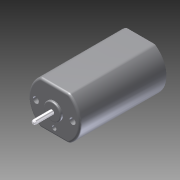
# Autodesk Inventor part: QFK-N30QAV-16068
Saved by Autodesk Inventor 2013 (Build 170138000, 138)
## iProperties
Category: Motoors
Company: Autodesk Inc.
Created: 2012-01-24
Part Number: QFK-N30QAV-16068
Material: Generic
Document SubType Name: Modeling
Designer: Autodesk Inc.
Density: 1 g/cm^3
Catalog Web Link: http://www.vexrobotics.com/276-2181.html
Vendor: VEX
Author: Autodesk Inc.
Autodesk Inventor part; units mm, degrees
ref_plane "YZ Plane" through (0, 0, 0) normal (1, 0, 0) x (0, 1, 0)
ref_plane "XZ Plane" through (0, 0, 0) normal (0, 1, 0) x (-1, 0, 0)
ref_plane "XY Plane" through (0, 0, 0) normal (0, 0, 1) x (1, 0, 0)
sketch "Sketch1" plane through (0, 0, 0) normal (0, 0, 1) x (1, 0, 0)
  line L0 (-3.0031, 5) -> (3.0031, 5)
  arc A0 (-3.597, 4.8023) -> (-3.6, -4.8) centre (0, 0) ccw
  line L1 (3.0031, -5) -> (-3.0031, -5)
  arc A1 (-3.597, 4.8023) -> (-3.597, -4.8023) centre (0, 0) ccw
  arc A2 (3.597, -4.8023) -> (3.597, 4.8023) centre (0, 0) ccw
  arc A3 (-3.0031, 5) -> (-3.597, 4.8023) centre (-3.0031, 4.0094) ccw
  arc A4 (3.597, 4.8023) -> (3.0031, 5) centre (3.0031, 4.0094) ccw
  arc A5 (3.0031, -5) -> (3.597, -4.8023) centre (3.0031, -4.0094) ccw
  arc A6 (-3.597, -4.8023) -> (-3.0031, -5) centre (-3.0031, -4.0094) ccw
  point P0 (0, 0)
  point P1 (3.3166, 5)
  point P2 (3.3166, -5)
  point P3 (-3.3166, -5)
  dimension "d0" = 0.9906
  constraints: 18 point on circle, 8 tangent, 7 centre point, 4 end point, 3 equal radius, 3 point on line
  measures "d0" radius of A3
extrude "Extrusion1" add sketch "Sketch1" along normal mid plane 19.9898
fillet "Fillet1" radius 0.508 8 edges at (-3.3161, 4.9493, 9.9949) (-6, 0, 9.9949) (-3.3161, -4.9493, 9.9949) (0, -5, 9.9949) (3.3161, -4.9493, 9.9949) (6, 0, 9.9949) (3.3161, 4.9493, 9.9949) (0, 5, 9.9949)
sketch "Sketch2" plane through (0, 0, 9.9949) normal (0, 0, 1) x (1, 0, 0)
  arc A0 (-3, 4.5) -> (-3.3, 4.4) centre (-2.9981, 3.9944) ccw
  spline S0 degree 3 poles (-3.3, 4.4) (-3.4685, 4.2736) (-3.6287, 4.1385) (-3.7806, 3.9947) (-3.8945, 3.8869) (-4.0038, 3.7742) (-4.1084, 3.6566) (-4.1433, 3.6174) (-4.1767, 3.5788) (-4.2115, 3.5374) (-4.4897, 3.2063) (-4.726, 2.8465) (-4.9194, 2.4597) (-5.0886, 2.1212) (-5.2214, 1.7694) (-5.3178, 1.4041) (-5.3315, 1.3519) (-5.3449, 1.298) (-5.3568, 1.2467) (-5.4522, 0.837) (-5.5, 0.4207) (-5.5, 0) (-5.5, -0.3681) (-5.4635, -0.7323) (-5.3904, -1.0926) (-5.38, -1.144) (-5.3691, -1.1941) (-5.3568, -1.2467) (-5.2588, -1.6679) (-5.1127, -2.0729) (-4.9194, -2.4597) (-4.7502, -2.7981) (-4.5484, -3.1155) (-4.3139, -3.4117) (-4.2805, -3.4541) (-4.2453, -3.4972) (-4.2115, -3.5374) (-3.941, -3.8595) (-3.6373, -4.147) (-3.3, -4.4) knots 0 0 0 0 0.0625 0.0625 0.0625 0.109375 0.109375 0.109375 0.125 0.125 0.125 0.25 0.25 0.25 0.359375 0.359375 0.359375 0.375 0.375 0.375 0.5 0.5 0.5 0.609375 0.609375 0.609375 0.625 0.625 0.625 0.75 0.75 0.75 0.859375 0.859375 0.859375 0.875 0.875 0.875 1 1 1 1
  arc A1 (-3.3, -4.4) -> (-3, -4.5) centre (-2.9981, -3.9944) ccw
  line L0 (-3, -4.5) -> (3, -4.5)
  arc A2 (3, -4.5) -> (3.3, -4.4) centre (2.9981, -3.9944) ccw
  arc A3 (3.3, -4.4) -> (3.3, 4.4) centre (0, 0) ccw
  arc A4 (3.3, 4.4) -> (3, 4.5) centre (2.9981, 3.9944) ccw
  line L1 (3, 4.5) -> (-3, 4.5)
  circle A5 centre (-4.25, 0) radius 0.7
  circle A6 centre (4.25, 0) radius 0.7
  circle A7 centre (0, 0) radius 2
  circle A8 centre (0, -3.5) radius 0.5
  circle A9 centre (0, -3.5) radius 0.5
  circle A10 centre (-4.25, 0) radius 0.7
  circle A11 centre (4.25, 0) radius 0.7
  circle A12 centre (0, 0) radius 2
  line L2 (3, 4.5) -> (-3, 4.5)
  arc A13 (-3, 4.5) -> (-3.3, 4.4) centre (-2.9981, 3.9944) ccw
  spline S1 degree 3 poles (-3.3, 4.4) (-3.4685, 4.2736) (-3.6287, 4.1385) (-3.7806, 3.9947) (-3.8945, 3.8869) (-4.0038, 3.7742) (-4.1084, 3.6566) (-4.1433, 3.6174) (-4.1767, 3.5788) (-4.2115, 3.5374) (-4.4897, 3.2063) (-4.726, 2.8465) (-4.9194, 2.4597) (-5.0886, 2.1212) (-5.2214, 1.7694) (-5.3178, 1.4041) (-5.3315, 1.3519) (-5.3449, 1.298) (-5.3568, 1.2467) (-5.4522, 0.837) (-5.5, 0.4207) (-5.5, 0) (-5.5, -0.3681) (-5.4635, -0.7323) (-5.3904, -1.0926) (-5.38, -1.144) (-5.3691, -1.1941) (-5.3568, -1.2467) (-5.2588, -1.6679) (-5.1127, -2.0729) (-4.9194, -2.4597) (-4.7502, -2.7981) (-4.5484, -3.1155) (-4.3139, -3.4117) (-4.2805, -3.4541) (-4.2453, -3.4972) (-4.2115, -3.5374) (-3.941, -3.8595) (-3.6373, -4.147) (-3.3, -4.4) knots 0 0 0 0 0.0625 0.0625 0.0625 0.109375 0.109375 0.109375 0.125 0.125 0.125 0.25 0.25 0.25 0.359375 0.359375 0.359375 0.375 0.375 0.375 0.5 0.5 0.5 0.609375 0.609375 0.609375 0.625 0.625 0.625 0.75 0.75 0.75 0.859375 0.859375 0.859375 0.875 0.875 0.875 1 1 1 1
  arc A14 (-3.3, -4.4) -> (-3, -4.5) centre (-2.9981, -3.9944) ccw
  line L3 (-3, -4.5) -> (3, -4.5)
  arc A15 (3, -4.5) -> (3.3, -4.4) centre (2.9981, -3.9944) ccw
  arc A16 (3.3, -4.4) -> (3.3, 4.4) centre (0, 0) ccw
  arc A17 (3.3, 4.4) -> (3, 4.5) centre (2.9981, 3.9944) ccw
  line L4 (-3, 5) -> (3, 5)
  arc A18 (3.6, -4.8) -> (3.6, 4.8) centre (0, 0) ccw
  arc A19 (-3.6, 4.8) -> (-3.6, -4.8) centre (0, 0) ccw
  line L5 (3, -5) -> (-3, -5)
  arc A20 (-3, 5) -> (-3.6, 4.8) centre (-3, 4) ccw
  constraints: 26 point on circle, 21 centre point, 12 end point, 4 other
extrude "Extrusion2" add sketch "Sketch2" along normal blind 0.508 contours A7
fillet "Fillet2" radius 0.254 1 edges at (-2, 0, 10.5029)
extrude "Extrusion3" cut sketch "Sketch2" against normal blind 2.9972 contours A5 | A6 | A8
sketch "Sketch3" plane through (0, 0, 10.5029) normal (0, 0, 1) x (1, 0, 0)
  circle A0 centre (0, 0) radius 1.746 projected
  circle A1 centre (0, 0) radius 0.4953
  dimension "d9" = 0.9906
  constraints: 1 centre point, 1 coincident
  measures "d9" diameter of A1
extrude "Extrusion4" add sketch "Sketch3" along normal blind 4.4958 contours A1
fillet "Fillet3" radius 0.4953 1 edges at (-0.4953, 0, 14.9987)
sketch "Sketch4" plane through (0, 0, -9.9949) normal (0, 0, -1) x (-1, 0, 0)
  arc A0 (-3.597, 4.8023) -> (-3.597, -4.8023) centre (0, 0) ccw projected
  circle A1 centre (0, 0) radius 2.5019
  dimension "d13" = 5.0038
  constraints: 1 centre point, 1 coincident
  measures "d13" diameter of A1
extrude "Extrusion5" add sketch "Sketch4" along normal blind 1.1938
sketch "Sketch5" plane through (0, 0, -9.9949) normal (0, 0, -1) x (-1, 0, 0)
  arc A0 (-3, 5) -> (-3.6, 4.8) centre (-3, 4) ccw
  arc A1 (-3.6, 4.8) -> (-3.6, -4.8) centre (0, 0) ccw
  arc A2 (-3.6, -4.8) -> (-3, -5) centre (-3, -4) ccw
  line L0 (3, -5) -> (-3, -5)
  arc A3 (3, -5) -> (3.6, -4.8) centre (3, -4) ccw
  arc A4 (3.6, -4.8) -> (3.6, 4.8) centre (0, 0) ccw
  arc A5 (3.6, 4.8) -> (3, 5) centre (3, 4) ccw
  line L1 (-3, 5) -> (3, 5)
  line L2 (3.7, -1.0714) -> (3.7, 1.0714)
  line L3 (3.4, -1.0714) -> (3.7, -1.0714)
  line L4 (3.4, 1.0714) -> (3.4, -1.0714)
  line L5 (3.7, 1.0714) -> (3.4, 1.0714)
  circle A6 centre (0, 0) radius 2.5
  line L6 (-3.7, -1.0714) -> (-3.4, -1.0714)
  line L7 (-3.7, 1.0714) -> (-3.7, -1.0714)
  line L8 (-3.4, 1.0714) -> (-3.7, 1.0714)
  line L9 (-3.4, -1.0714) -> (-3.4, 1.0714)
  constraints: 20 end point, 12 point on circle, 7 centre point
extrude "Extrusion6" add sketch "Sketch5" along normal blind 1.6002 contours L3 L4 L5 L2 | L7 L8 L9 L6
chamfer "Chamfer1" distance 0.508 angle 45 4 edges at (3.55, 1.0714, -11.5951) (3.55, -1.0714, -11.5951) (-3.55, 1.0714, -11.5951) (-3.55, -1.0714, -11.5951)
body "Solid1"
